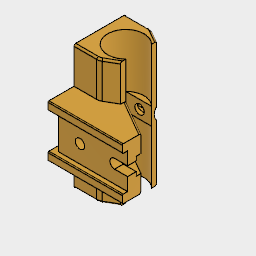
Z_Axis_Bearing_Holder_1.0_F01 (Autodesk Fusion 360 design; units mm, degrees)
Autodesk Fusion 360 part; units mm, degrees
sketch "スケッチ1" plane through (0, 0, 0) normal (0, 0, 1) x (1, 0, 0)
  circle A0 centre (0, 0) radius 10.5
  line L0 (-15, 15) -> (-15, -15)
  line L1 (-15, -15) -> (-0.5, -15)
  line L2 (-0.5, -15) -> (7.425, -10.4245)
  line L3 (7.425, -10.4245) -> (7.425, 10.4245)
  line L4 (7.425, 10.4245) -> (-0.5, 15)
  line L5 (-0.5, 15) -> (-15, 15)
  line L6 (7.425, 7.4242) -> (-7.425, 7.4242)
  dimension "d1" = 21
  dimension "d2" = 15
  dimension "d3" = 30
  dimension "d4" = 15
  dimension "d5" = 22.425
  dimension "d6" = 150
  dimension "d7" = 150
  dimension "d8" = 14.5
  dimension "d9" = 14.5
  measures "d1" diameter of A0
  measures "d2" distance of A0.centre L0
  measures "d3" distance of L1 L5
  measures "d4" distance of A0.centre L5
  measures "d5" distance of L0 L3
  measures "d6" angle of L1 L2
  measures "d7" angle of L4 L5
  measures "d8" distance of L0.end L1.end
  measures "d9" distance of L0.start L4.end
extrude "押し出し1" add sketch "スケッチ1" along normal mid plane 72 contours A0 L0 L1 L2 L3 L4 L5
extrude "押し出し9" add sketch "スケッチ1" along normal mid plane 10 contours A0 L6
sketch "スケッチ2" plane through (0, 0, 0) normal (0, 0, 1) x (1, 0, 0)
  line L0 (-15, -15) -> (-15, -30)
  line L1 (-15, -30) -> (28, -30)
  line L2 (28, -30) -> (28, -7.4242)
  line L3 (28, -7.4242) -> (7.425, -7.4242)
  line L4 (7.425, -7.4242) -> (7.425, -10.4245)
  line L5 (7.425, -10.4245) -> (-0.5, -15)
  line L6 (7.425, -10.4245) -> (-0.5, -15)
  line L7 (-15, -15) -> (-0.5, -15)
  line L8 (7.425, -7.4242) -> (28, -19.304)
  line L9 (-0.5, 15) -> (-15, 15)
  line L10 (-15, 15) -> (-15, 19.5)
  line L11 (-15, 19.5) -> (-8.2942, 19.5)
  line L12 (-8.2942, 19.5) -> (-0.5, 15)
  line L13 (7.425, 10.4245) -> (-0.5, 15)
  point P0 (-15, -15)
  point P1 (7.425, -7.4242)
  point P2 (7.425, -10.4245)
  point P3 (-0.5, -15)
  point P4 (-15, 15)
  dimension "d12" = 43
  dimension "d13" = 30
  dimension "d14" = 10.696
  dimension "d15" = 4.5
  measures "d12" distance of L0 L2
  measures "d13" distance of origin L1
  measures "d14" distance of L1.end L8.end
  measures "d15" distance of L9 L11
extrude "押し出し2" add sketch "スケッチ2" along normal mid plane 30 contours L0 L1 L2 L4 L5 L6 L7 L8 | L9 L10 L11 L12
sketch "スケッチ3" plane through (28, 0, 0) normal (1, 0, 0) x (0, 1, 0)
  line L0 (-19.304, -15) -> (-19.304, 15)
  line L1 (-19.304, 15) -> (-30, 15)
  line L2 (-30, 15) -> (-30, -15)
  line L3 (-30, -15) -> (-19.304, -15)
  line L4 (-30, 10.2) -> (-27, 10.2)
  line L5 (-27, 10.2) -> (-27, -10.2)
  line L6 (-27, -10.2) -> (-30, -10.2)
  line L7 (-7.4242, -15) -> (-7.4242, 15)
  line L8 (-7.4242, 5) -> (-22, 5)
  line L9 (-22, 5) -> (-22, -5)
  line L10 (-22, -5) -> (-7.4242, -5)
  dimension "d18" = 3
  dimension "d19" = 20.4
  dimension "d20" = 10.2
  dimension "d21" = 5
  dimension "d22" = 10
  dimension "d23" = 5
  measures "d18" distance of L2 L5
  measures "d19" distance of L4 L6
  measures "d20" distance of origin L4
  measures "d21" distance of L5 L9
  measures "d22" distance of L8 L10
  measures "d23" distance of origin L8
sketch "スケッチ4" plane through (0, 19.5, 0) normal (0, 1, 0) x (-1, 0, 0)
  line L0 (15, -15) -> (15, 15)
  line L1 (15, 15) -> (8.2942, 15)
  line L2 (8.2942, 15) -> (8.2942, -15)
  line L3 (8.2942, -15) -> (15, -15)
  line L4 (15, 10.2) -> (12, 10.2)
  line L5 (12, 10.2) -> (12, -10.2)
  line L6 (12, -10.2) -> (15, -10.2)
  dimension "d24" = 3
  dimension "d25" = 20.4
  dimension "d26" = 10.2
  measures "d24" distance of L0 L5
  measures "d25" distance of L4 L6
  measures "d26" distance of origin L4
extrude "押し出し3" cut sketch "スケッチ3" against normal up to surface (43 mm away) contours L2 L4 L5 L6
extrude "押し出し4" cut sketch "スケッチ4" against normal up to surface (46.5 mm away) contours L0 L4 L5 L6
extrude "押し出し5" cut sketch "スケッチ3" against normal blind 35 contours L0 L8 L9 L10 | L0 L7 L8 L10
ref_plane "作業平面1" through (-7.5, 0, 0) normal (1, 0, 0) x (0, 1, 0)
sketch "スケッチ5" plane through (-7.5, 0, 0) normal (1, 0, 0) x (0, 1, 0)
  circle A0 centre (14, 0) radius 5
  circle A1 centre (14, 0) radius 2.7
  line L0 (19.5, 15) -> (19.5, -15)
  line L1 (15, 15) -> (19.5, 15)
  line L2 (7.4242, -5) -> (7.4242, -36)
  line L3 (7.4242, 5) -> (19.5, 5)
  line L4 (7.4242, -5) -> (19.5, -5)
  line L5 (10.4242, 5) -> (10.4242, -5)
  line L6 (7.4242, 36) -> (7.4242, 5)
  dimension "d38" = 10
  dimension "d39" = 5.4
  dimension "d40" = 5.5
  dimension "d41" = 15
  dimension "d42" = 3
  measures "d38" diameter of A0
  measures "d39" diameter of A1
  measures "d40" distance of A0.centre L0
  measures "d41" distance of A0.centre L1
  measures "d42" distance of L2 L5
extrude "押し出し7" cut sketch "スケッチ5" along normal blind 20 contours A0 L5 | A0 L0 L3 L4 | A0 L5 | A1
extrude "押し出し8" cut sketch "スケッチ5" against normal blind 10 contours A1
sketch "スケッチ6" plane through (-12, 0, 0) normal (-1, 0, 0) x (0, -1, 0)
  circle A0 centre (-14, 0) radius 2.7
  line L0 (27, -10.2) -> (27, 10.2)
  line L1 (27, 10.2) -> (-19.5, 10.2)
  line L2 (-19.5, 10.2) -> (-19.5, -10.2)
  line L3 (-19.5, -10.2) -> (27, -10.2)
  line L4 (17, 10.2) -> (17, -10.2) construction
  circle A1 centre (17, 0) radius 2.7
  dimension "d56" = 10
  dimension "d57" = 5.4
  measures "d56" distance of L0 L4
  measures "d57" diameter of A1
extrude "押し出し10" cut sketch "スケッチ6" against normal up to surface (5 mm away) contours A1
sketch "スケッチ7" plane through (0, -27, 0) normal (0, -1, 0) x (1, 0, 0)
  line L0 (-12, 10.2) -> (-12, -10.2)
  line L1 (-12, -10.2) -> (28, -10.2)
  line L2 (28, -10.2) -> (28, 10.2)
  line L3 (28, 10.2) -> (-12, 10.2)
  circle A0 centre (0.5, 0) radius 2.7
  line L4 (-12, 0) -> (0.5, 0) construction
  line L5 (28, 0) -> (20.5, 0) construction
  circle A1 centre (20.5, 0) radius 2.7
  line L6 (28, 2.7) -> (20.5, 2.7)
  line L7 (28, -2.7) -> (20.5, -2.7)
  point P0 (-12, 0)
  dimension "d60" = 5.4
  dimension "d61" = 12.5
  dimension "d64" = 7.5
  dimension "d65" = 5.4
  measures "d60" diameter of A0
  measures "d61" distance of P0 A0.centre
  measures "d64" distance of L5.start L5.end
  measures "d65" diameter of A1
extrude "押し出し11" cut sketch "スケッチ7" against normal blind 40 contours A0
extrude "押し出し12" cut sketch "スケッチ7" against normal blind 5 contours L2 A1 L6 L7 | A1
fillet "フィレット1" radius 5 5 edges at (-0.5, 15, 25.5) (-8.2942, 19.5, 0) (-0.5, 15, -25.5) (-0.5, -15, -25.5) (-0.5, -15, 25.5)
fillet "フィレット2" radius 1 20 edges at (-8.4199, -15, 36) (-0.5457, -14.8296, 36) (4.0426, -12.3773, 36) (4.0426, 12.3773, 36) (-0.5457, 14.8296, 36) (-8.4199, 15, 36) (-3.2369, 16.5801, 15) (-8.3399, 19.3296, 15) (-12.317, 19.5, 15) (-12.317, 19.5, -15) (-8.3399, 19.3296, -15) (-3.2369, 16.5801, -15) (-8.4199, 15, -36) (-0.5457, 14.8296, -36) (4.0426, 12.3773, -36) (4.0426, -12.3773, -36) (-0.5457, -14.8296, -36) (-8.4199, -15, -36) (17.7125, -13.3641, -15) (17.7125, -13.3641, 15)
fillet "フィレット3" radius 0.5 4 edges at (6.5, -30, 15) (6.5, -30, 10.2) (6.5, -30, -10.2) (6.5, -30, -15)
equation "d4 = d3 / 2"
equation "d9 = d8"
equation "d20 = d19 / 2"
equation "d23 = d22 / 2"
equation "d26 = d25 / 2"
